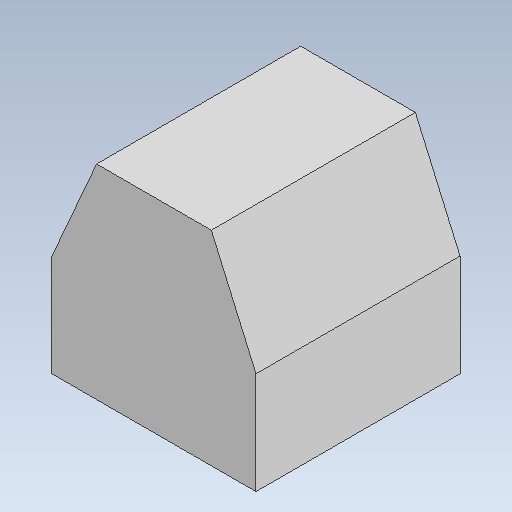
# Autodesk Inventor part: tooth
Saved by Autodesk Inventor 2021 (Build 250183000, 183)
## iProperties
Created: 2021-05-05
Part Number: tooth
Material: Generic
Document SubType Name: Modeling
Density: 1 g/cm^3
Appearance: Default
Autodesk Inventor part; units mm, degrees
ref_plane "YZ Plane" through (0, 0, 0) normal (1, 0, 0) x (0, 1, 0)
ref_plane "XZ Plane" through (0, 0, 0) normal (0, 1, 0) x (-1, 0, 0)
ref_plane "XY Plane" through (0, 0, 0) normal (0, 0, 1) x (1, 0, 0)
sketch "Sketch1" plane through (0, 0, 0) normal (0, 0, 1) x (1, 0, 0)
  line L0 (-5, -2.6054) -> (-5, 2.3946)
  line L1 (-5, -2.6054) -> (0, -2.6054)
  line L2 (0, -2.6054) -> (0, 7.3946)
  line L3 (0, 7.3946) -> (-2.8105, 7.3946)
  line L4 (-2.8105, 7.3946) -> (-5, 2.3946)
  point P0 (0, 0)
  dimension "d0" = 5
  dimension "d1" = 5
  dimension "d2" = 5
  constraints: 10 end point, 2 horizontal, 1 perpendicular, 1 point on line, 1 vertical
  measures "d0" distance of L0.start L0.end
  measures "d1" distance from line of L3 L0.end
  measures "d2" distance of L0.start L1.end
extrude "Extrusion1" add sketch "Sketch1" along normal blind 10
mirror "Mirror1" about plane through (0, 0, 0) normal (1, 0, 0) of "Extrusion1"
equation "\"d0\" = rack_tooth_dedendum"
equation "\"d1\" = rack_tooth_addendum"
equation "\"d2\" = rack_tooth_thickness"
equation "\"d3\" = rack_tooth_face_widh"
equation "\"rack_tooth_thickness\" = 5"
equation "\"rack_tooth_face_widh\" = 10"
equation "\"rack_tooth_addendum\" = 5"
equation "\"rack_tooth_dedendum\" = 5"
equation "\"secure_arm_angle\" = 20deg"
equation "\"secure_arm_radii\" = 9"
equation "\"hoop_bearing_length\" = 5deg"
equation "\"secure_arm_hold_length\" = 35"
equation "\"hoop_cable_pulley_diam\" = 22"
equation "\"hoop_cable_diam\" = 5"
equation "\"support_frame_squareBarThickness\" = 5"
equation "\"support_frame_squareBarFillet\" = 2"
equation "\"support_baseClamp_platformThickness\" = 15"
equation "\"support_baseClamp_platformWidthBuffer\" = 0"
equation "\"support_baseClamp_platformLengthBuffer\" = 35"
equation "\"support_frame_endHoleBuffer\" = 25"
equation "\"support_baseClamp_thickness\" = 8"
equation "\"support_baseClamp_sleeveSweepTerminationAngle\" = 55deg"
equation "\"support_baseClamp_sleeveHoleDiameter\" = 12"
equation "\"hoop_angle_z\" = 45deg"
body "Solid1"
